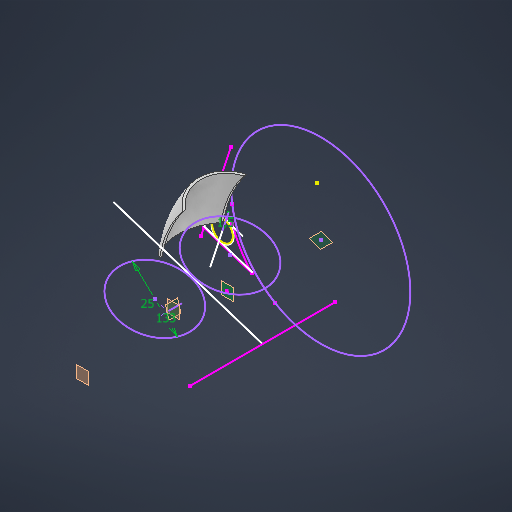
# Autodesk Inventor part: подьем колеса 25-26
Saved by Autodesk Inventor 2025 (Build 290162000, 162)
## iProperties
Created: 2025-10-03
Part Number: подьем колеса 25-26
Material: Типовые
Document SubType Name: Modeling
Designer: Phantom
Density: 1 g/cm^3
Appearance: По умолчанию
Author: Phantom
Autodesk Inventor part; units mm, degrees
ref_plane "YZ Plane" through (0, 0, 0) normal (1, 0, 0) x (0, 1, 0)
ref_plane "XZ Plane" through (0, 0, 0) normal (0, 1, 0) x (-1, 0, 0)
ref_plane "XY Plane" through (0, 0, 0) normal (0, 0, 1) x (1, 0, 0)
ref_plane "РабПлоскость15" through (0, 0, 121) normal (0, 0, -1) x (-1, 0, 0)
sketch "Эскиз13" plane through (0, 0, 121) normal (0, 0, -1) x (-1, 0, 0)
  arc A0 (18.116, 75.0583) -> (12.6723, 73.0313) centre (8.93, 91.404) ccw projected
  arc A1 (15.1818, 72.1432) -> (12.9717, 71.5614) centre (8.93, 91.404) ccw
  line L0 (8.93, 91.404) -> (31.1796, 22.8568)
  line L1 (42.9225, 78.788) -> (48.2834, 62.2719) projected
  line L2 (8.93, 91.404) -> (-2.0706, 125.2951)
  line L3 (28.8205, 122.2337) -> (-9.1771, 109.9002) projected
  line L4 (-44.1807, 50.678) -> (42.9225, 78.788) projected
  line L5 (-6.3666, 230.6392) -> (28.8205, 122.2337) projected
  line L6 (28.8205, 122.2337) -> (42.9225, 78.788)
  line L7 (-27.6965, 100.8055) -> (34.3413, 120.9422)
  line L8 (-44.935, 52.7423) -> (51.7275, 83.9372)
  arc A2 (-44.1807, 50.678) -> (-9.1771, 109.9002) centre (-170, 165) ccw projected
  point P0 (0, 0)
  point P1 (1.7728, 113.4543)
  point P2 (2.6782, 110.6648)
  point P3 (15.8599, 70.0544)
  point P4 (-10.4135, 106.4154)
  point P5 (2.6782, 110.6648)
  point P6 (-41.3188, 53.9093)
  point P7 (15.1818, 72.1432)
  dimension "d40" = 1.5
  constraints: 10 end point, 3 parallel, 2 point on circle, 2 tangent, 1 centre point, 1 point on line
  measures "d40" radial gap between concentric circles of A0 A1
ref_plane "РабПлоскость11" through (0, 0, 385) normal (0, 0, 1) x (1, 0, 0)
sketch "Эскиз17" plane through (0, 0, 385) normal (0, 0, 1) x (1, 0, 0)
  arc A0 (8.2707, 230.0212) -> (8.6956, 141.5501) centre (165.364, 186.5392) ccw projected
  line L0 (165.364, 186.5392) -> (8.6956, 141.5501)
  point P0 (0, 0)
  constraints: 2 end point, 1 coincident
ref_plane "РабПлоскость2" through (165.364, 186.5392, 385) normal (-0.9611557, -0.2760066, 0) x (0.2760066, -0.9611557, 0)
ref_plane "РабПлоскость3" through (165.364, 186.5392, 385) normal (0, 0, 1) x (1, 0, 0)
sketch "Эскиз18" plane through (165.364, 186.5392, 385) normal (0, 0, 1) x (1, 0, 0)
  circle A0 centre (0, 0) radius 163
  line L0 (0, 0) -> (-156.6684, -44.9891) projected
  circle A1 centre (-95.635, -27.4627) radius 63.5
  point P0 (-165.364, -186.5392)
  dimension "d55" = 127
  constraints: 1 centre point, 1 coincident, 1 point on line, 3 other
  measures "d55" diameter of A1
ref_plane "РабПлоскость4" through (69.729, 159.0765, 385) normal (-0.9611557, -0.2760066, 0) x (0.2760066, -0.9611557, 0)
sketch "Эскиз19" plane through (69.729, 159.0765, 385) normal (-0.9611557, -0.2760066, 0) x (0.2760066, -0.9611557, 0)
  line L0 (0, 0) -> (0, -127)
  line L1 (0, -40) -> (0, 0) projected
  ellipse E0 centre (0, -63.5) end of major axis (0, 0) minor radius 63.5
  point P0 (133.6516, -385)
  dimension "d57" = 63.5
  dimension "d56" = 127
  constraints: 2 end point, 2 vertical, 1 midpoint, 1 vertical alignment, 2 other
  measures "d56" distance of L0.start L0.end
ref_plane "РабПлоскость6" through (8.6956, 141.5501, 121) normal (-0.3087313, -0.9511493, 0) x (0.9511493, -0.3087313, 0)
ref_plane "РабПлоскость14" through (0, 0, 121) normal (0, 0, -1) x (-1, 0, 0)
sketch "Эскиз20" plane through (8.6956, 141.5501, 121) normal (-0.3087313, -0.9511493, 0) x (0.9511493, -0.3087313, 0)
  circle A0 centre (62.6409, 200.5) radius 66.5
  line L0 (196.9671, 0) -> (196.9671, 264) projected
  line L1 (196.9671, 132) -> (-88.0095, 132)
  circle A1 centre (62.6409, 63.5) radius 66.5
  line L2 (87.6409, 200.5) -> (87.6409, 175.2953)
  point P0 (35.4301, -121)
  dimension "d58" = 133
  dimension "d72" = 25
  constraints: 4 end point, 2 centre point, 1 coincident, 1 horizontal, 1 midpoint, 1 symmetric about line, 1 vertical, 1 other
  measures "d58" diameter of A0
  measures "d72" distance of A0.centre L2.start
sketch "Эскиз21" plane through (0, 0, 121) normal (0, 0, -1) x (-1, 0, 0)
  arc A0 (-86.2538, 25.1587) -> (-8.6956, 141.5501) centre (-170, 165) ccw projected
  circle A1 centre (-170, 165) radius 163
  point P0 (0, 0)
  constraints: 1 centre point, 1 coincident, 1 concentric
ref_plane "РабПлоскость16" through (0, 0, 385) normal (0, 0, 1) x (1, 0, 0)
ref_plane "РабПлоскость23" through (170, 165, 121) normal (-0.3087313, -0.9511493, 0) x (0.9511493, -0.3087313, 0)
sketch "Эскиз42" plane through (170, 165, 121) normal (-0.3087313, -0.9511493, 0) x (0.9511493, -0.3087313, 0)
  line L0 (-146.1848, 0) -> (-36.4817, 0) projected
  line L1 (-163, 0) -> (163, 0) projected
  circle A0 centre (-83.5439, 63.5) radius 66.5 projected
  line L2 (-83.5439, 63.5) -> (-213.4918, 63.5)
  line L3 (-163, 0) -> (-163, 105.851)
  circle A1 centre (-96.5, 63.5) radius 66.5
  circle A2 centre (-96.5, 63.5) radius 70.5
  line L4 (-136, 121.8952) -> (-136, -30.0897)
  line L5 (0, 0) -> (0, 130)
  point P0 (-110.7547, -121)
  point P1 (-136, 116.9977)
  point P2 (-136, 5.1048)
  point P3 (-136, 10.0023)
  point P4 (-167, 63.5)
  dimension "d132" = 133
  dimension "d133" = 141
  dimension "d135" = 31
  constraints: 8 end point, 3 vertical, 2 centre point, 2 point on circle, 2 point on line, 1 coincident, 1 horizontal, 1 midpoint, 1 tangent
  measures "d132" diameter of A1
  measures "d133" diameter of A2
  measures "d135" distance from line of A2.end L4
revolve "Вращение1" add sketch "Эскиз42" angle 30 about axis through (196.0408, 80.7402, 121) along (0, 0, 1) contours A2 L3 A1 L4 | A2 L2 L3 | L2 A2 L3 | L3 A2 L4 A1
